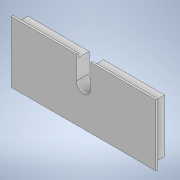
# Autodesk Inventor part: PrintHeadCap
Saved by Autodesk Inventor 2021 (Build 250183000, 183)
## iProperties
Created: 2022-02-21
Part Number: PrintHeadCap
Material: Generic
Document SubType Name: Sheet Metal
Designer: Unit-005
Density: 1 g/cm^3
Sheet Metal Rule: Default
Appearance: Default
Author: Unit-005
## iProperties of the stored document _3DPrint.ipt
Created: 2022-02-21
Part Number: _3DPrint
Material: Generic
Document SubType Name: Modeling
Designer: Unit-005
Density: 1 g/cm^3
Appearance: Default
Author: Unit-005
Autodesk Inventor part; units mm, degrees
ref_plane "YZ Plane" through (0, 0, 0) normal (1, 0, 0) x (0, 1, 0)
ref_plane "XZ Plane" through (0, 0, 0) normal (0, 1, 0) x (-1, 0, 0)
ref_plane "XY Plane" through (0, 0, 0) normal (0, 0, 1) x (1, 0, 0)
sketch "Sketch1" plane through (0, 0, 0) normal (0, 0, 1) x (1, 0, 0)
  line L0 (-18.875, 7.375) -> (18.875, 7.375)
  line L1 (18.875, 7.375) -> (18.875, -7.375)
  line L2 (18.875, -7.375) -> (-18.875, -7.375)
  line L3 (-18.875, -7.375) -> (-18.875, 7.375)
  line L4 (-18.875, 7.375) -> (18.875, -7.375) construction
  line L5 (18.875, 7.375) -> (-18.875, -7.375) construction
  point P0 (0, 0)
  dimension "d0" = 37.75
  dimension "d1" = 14.75
  constraints: 12 end point, 2 midpoint, 2 parallel, 1 horizontal, 1 perpendicular
  measures "d0" distance of L1.end L2.end
  measures "d1" distance of L0.end L1.end
extrude "Extrusion1" add sketch "Sketch1" along normal blind 3
sketch "Sketch2" plane through (0, 0, 3) normal (0, 0, 1) x (1, 0, 0)
  line L0 (-18.875, -7.375) -> (18.875, -7.375) projected
  line L1 (18.875, -7.375) -> (18.875, 7.375) projected
  line L2 (18.875, 7.375) -> (-18.875, 7.375) projected
  line L3 (-18.875, 7.375) -> (-18.875, -7.375) projected
  line L4 (-20, 8.5) -> (20, 8.5)
  line L5 (20, 8.5) -> (20, -8.5)
  line L6 (20, -8.5) -> (-20, -8.5)
  line L7 (-20, -8.5) -> (-20, 8.5)
  line L8 (-20, 8.5) -> (20, -8.5) construction
  line L9 (20, 8.5) -> (-20, -8.5) construction
  point P0 (0, 0)
  dimension "d4" = 40
  dimension "d5" = 17
  constraints: 12 end point, 2 midpoint, 2 parallel, 1 horizontal, 1 perpendicular
  measures "d4" distance of L5.end L6.end
  measures "d5" distance of L4.end L5.end
extrude "Extrusion2" add sketch "Sketch2" along normal blind 0.5 contours L3 L2 L1 L0 | L4 L5 L6 L7
sketch "Sketch3" plane through (0, 0, 3.5) normal (0, 0, 1) x (1, 0, 0)
  line L0 (-20, -8.5) -> (20, -8.5) projected
  line L1 (20, -8.5) -> (20, 8.5) projected
  line L2 (20, 8.5) -> (-20, 8.5) projected
  line L3 (-20, 8.5) -> (-20, -8.5) projected
  line L4 (20, 8.5) -> (-20, 8.5) projected
  line L5 (-2, 0) -> (2, 0)
  line L6 (2, 0) -> (2, 8.5)
  line L7 (2, 8.5) -> (-2, 8.5)
  line L8 (-2, 8.5) -> (-2, 0)
  line L9 (0, -11.9) -> (0, 11.9) projected
  line L10 (-28, 0) -> (28, 0) projected
  point P0 (0, 0)
  dimension "d8" = 4
  constraints: 8 end point, 2 parallel, 1 collinear, 1 horizontal, 1 perpendicular, 1 point on line, 1 other
  measures "d8" distance of L7.end L6.end
extrude "Extrusion3" cut sketch "Sketch3" against normal through all contours L9 L2 L6 L5 | L5 L8 L2 L9
fillet "Fillet1" radius 2 2 edges at (-2, 0, 1.75) (2, 0, 1.75)
equation "\"BendRadius\" = Thickness"
equation "\"BendReliefWidth\" = Thickness"
equation "\"BendReliefDepth\" = 0.5 * Thickness"
equation "\"CornerReliefSize\" = 4 * Thickness"
equation "\"MinimumRemnant\" = 2 * Thickness"
equation "\"TransitionRadius\" = BendRadius"
equation "\"JacobiRadiusSize\" = BendRadius"
equation "\"GapSize\" = Thickness"
equation "\"Thickness\" = 3.048"
body "Solid1"
